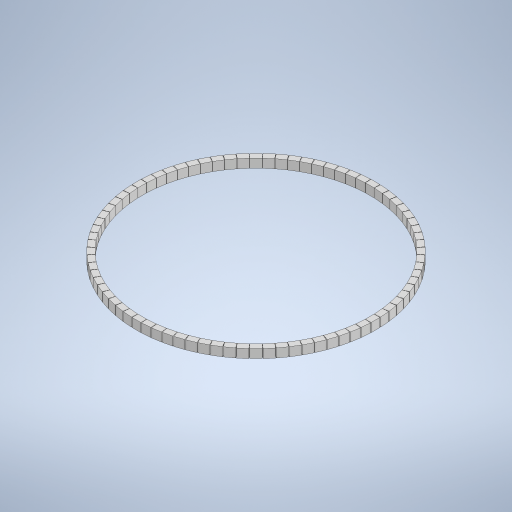
# Autodesk Inventor part: 屋-2 磚-1
Saved by Autodesk Inventor 2024 (Build 280153000, 153)
## iProperties
Created: 2024-05-21
Part Number: 屋-2 磚-1
Material: 一般
Document SubType Name: Modeling
Designer: User
Density: 1 g/cm^3
Appearance: 預設
Author: User
Autodesk Inventor part; units mm, degrees
ref_plane "YZ Plane" through (0, 0, 0) normal (1, 0, 0) x (0, 1, 0)
ref_plane "XZ Plane" through (0, 0, 0) normal (0, 1, 0) x (-1, 0, 0)
ref_plane "XY Plane" through (0, 0, 0) normal (0, 0, 1) x (1, 0, 0)
sketch "草圖1" plane through (0, 0, 0) normal (0, 1, 0) x (-1, 0, 0)
  circle A0 centre (0, 0) radius 20
  line L0 (19.5, 0.75) -> (20.5, 0.75)
  line L1 (20.5, 0.75) -> (20.5, -0.75)
  line L2 (20.5, -0.75) -> (19.5, -0.75)
  line L3 (19.5, -0.75) -> (19.5, 0.75)
  line L4 (19.5, 0.75) -> (20.5, -0.75) construction
  line L5 (20.5, 0.75) -> (19.5, -0.75) construction
  line L6 (20.378, 2.3561) -> (20.4956, 0.8607)
  line L7 (20.4956, 0.8607) -> (19.4987, 0.7823)
  line L8 (19.4987, 0.7823) -> (19.381, 2.2776)
  line L9 (19.381, 2.2776) -> (20.378, 2.3561)
  line L10 (20.1303, 3.9477) -> (20.3649, 2.4661)
  line L11 (20.3649, 2.4661) -> (19.3772, 2.3097)
  line L12 (19.3772, 2.3097) -> (19.1426, 3.7912)
  line L13 (19.1426, 3.7912) -> (20.1303, 3.9477)
  line L14 (19.7585, 5.5149) -> (20.1087, 4.0564)
  line L15 (20.1087, 4.0564) -> (19.1363, 3.8229)
  line L16 (19.1363, 3.8229) -> (18.7861, 5.2815)
  line L17 (18.7861, 5.2815) -> (19.7585, 5.5149)
  line L18 (19.2649, 7.0481) -> (19.7284, 5.6216)
  line L19 (19.7284, 5.6216) -> (18.7774, 5.3125)
  line L20 (18.7774, 5.3125) -> (18.3138, 6.7391)
  line L21 (18.3138, 6.7391) -> (19.2649, 7.0481)
  line L22 (18.6525, 8.5379) -> (19.2265, 7.1521)
  line L23 (19.2265, 7.1521) -> (18.3027, 6.7694)
  line L24 (18.3027, 6.7694) -> (17.7286, 8.1552)
  line L25 (17.7286, 8.1552) -> (18.6525, 8.5379)
  line L26 (17.9251, 9.9751) -> (18.6061, 8.6386)
  line L27 (18.6061, 8.6386) -> (17.7151, 8.1846)
  line L28 (17.7151, 8.1846) -> (17.0341, 9.5211)
  line L29 (17.0341, 9.5211) -> (17.9251, 9.9751)
  line L30 (17.0872, 11.3507) -> (17.871, 10.0717)
  line L31 (17.871, 10.0717) -> (17.0184, 9.5492)
  line L32 (17.0184, 9.5492) -> (16.2346, 10.8282)
  line L33 (16.2346, 10.8282) -> (17.0872, 11.3507)
  line L34 (16.144, 12.6564) -> (17.0257, 11.4428)
  line L35 (17.0257, 11.4428) -> (16.2167, 10.855)
  line L36 (16.2167, 10.855) -> (15.335, 12.0686)
  line L37 (15.335, 12.0686) -> (16.144, 12.6564)
  line L38 (15.1012, 13.884) -> (16.0754, 12.7434)
  line L39 (16.0754, 12.7434) -> (15.315, 12.0939)
  line L40 (15.315, 12.0939) -> (14.3408, 13.2345)
  line L41 (14.3408, 13.2345) -> (15.1012, 13.884)
  line L42 (13.9654, 15.026) -> (15.026, 13.9654)
  line L43 (15.026, 13.9654) -> (14.3189, 13.2583)
  line L44 (14.3189, 13.2583) -> (13.2583, 14.3189)
  line L45 (13.2583, 14.3189) -> (13.9654, 15.026)
  line L46 (12.7434, 16.0754) -> (13.884, 15.1012)
  line L47 (13.884, 15.1012) -> (13.2345, 14.3408)
  line L48 (13.2345, 14.3408) -> (12.0939, 15.315)
  line L49 (12.0939, 15.315) -> (12.7434, 16.0754)
  line L50 (11.4428, 17.0257) -> (12.6564, 16.144)
  line L51 (12.6564, 16.144) -> (12.0686, 15.335)
  line L52 (12.0686, 15.335) -> (10.855, 16.2167)
  line L53 (10.855, 16.2167) -> (11.4428, 17.0257)
  line L54 (10.0717, 17.871) -> (11.3507, 17.0872)
  line L55 (11.3507, 17.0872) -> (10.8282, 16.2346)
  line L56 (10.8282, 16.2346) -> (9.5492, 17.0184)
  line L57 (9.5492, 17.0184) -> (10.0717, 17.871)
  line L58 (8.6386, 18.6061) -> (9.9751, 17.9251)
  line L59 (9.9751, 17.9251) -> (9.5211, 17.0341)
  line L60 (9.5211, 17.0341) -> (8.1846, 17.7151)
  line L61 (8.1846, 17.7151) -> (8.6386, 18.6061)
  line L62 (7.1521, 19.2265) -> (8.5379, 18.6525)
  line L63 (8.5379, 18.6525) -> (8.1552, 17.7286)
  line L64 (8.1552, 17.7286) -> (6.7694, 18.3027)
  line L65 (6.7694, 18.3027) -> (7.1521, 19.2265)
  line L66 (5.6216, 19.7284) -> (7.0481, 19.2649)
  line L67 (7.0481, 19.2649) -> (6.7391, 18.3138)
  line L68 (6.7391, 18.3138) -> (5.3125, 18.7774)
  line L69 (5.3125, 18.7774) -> (5.6216, 19.7284)
  line L70 (4.0564, 20.1087) -> (5.5149, 19.7585)
  line L71 (5.5149, 19.7585) -> (5.2815, 18.7861)
  line L72 (5.2815, 18.7861) -> (3.8229, 19.1363)
  line L73 (3.8229, 19.1363) -> (4.0564, 20.1087)
  line L74 (2.4661, 20.3649) -> (3.9477, 20.1303)
  line L75 (3.9477, 20.1303) -> (3.7912, 19.1426)
  line L76 (3.7912, 19.1426) -> (2.3097, 19.3772)
  line L77 (2.3097, 19.3772) -> (2.4661, 20.3649)
  line L78 (0.8607, 20.4956) -> (2.3561, 20.378)
  line L79 (2.3561, 20.378) -> (2.2776, 19.381)
  line L80 (2.2776, 19.381) -> (0.7823, 19.4987)
  line L81 (0.7823, 19.4987) -> (0.8607, 20.4956)
  line L82 (-0.75, 20.5) -> (0.75, 20.5)
  line L83 (0.75, 20.5) -> (0.75, 19.5)
  line L84 (0.75, 19.5) -> (-0.75, 19.5)
  line L85 (-0.75, 19.5) -> (-0.75, 20.5)
  line L86 (-2.3561, 20.378) -> (-0.8607, 20.4956)
  line L87 (-0.8607, 20.4956) -> (-0.7823, 19.4987)
  line L88 (-0.7823, 19.4987) -> (-2.2776, 19.381)
  line L89 (-2.2776, 19.381) -> (-2.3561, 20.378)
  line L90 (-3.9477, 20.1303) -> (-2.4661, 20.3649)
  line L91 (-2.4661, 20.3649) -> (-2.3097, 19.3772)
  line L92 (-2.3097, 19.3772) -> (-3.7912, 19.1426)
  line L93 (-3.7912, 19.1426) -> (-3.9477, 20.1303)
  line L94 (-5.5149, 19.7585) -> (-4.0564, 20.1087)
  line L95 (-4.0564, 20.1087) -> (-3.8229, 19.1363)
  line L96 (-3.8229, 19.1363) -> (-5.2815, 18.7861)
  line L97 (-5.2815, 18.7861) -> (-5.5149, 19.7585)
  line L98 (-7.0481, 19.2649) -> (-5.6216, 19.7284)
  line L99 (-5.6216, 19.7284) -> (-5.3125, 18.7774)
  line L100 (-5.3125, 18.7774) -> (-6.7391, 18.3138)
  line L101 (-6.7391, 18.3138) -> (-7.0481, 19.2649)
  line L102 (-8.5379, 18.6525) -> (-7.1521, 19.2265)
  line L103 (-7.1521, 19.2265) -> (-6.7694, 18.3027)
  line L104 (-6.7694, 18.3027) -> (-8.1552, 17.7286)
  line L105 (-8.1552, 17.7286) -> (-8.5379, 18.6525)
  line L106 (-9.9751, 17.9251) -> (-8.6386, 18.6061)
  line L107 (-8.6386, 18.6061) -> (-8.1846, 17.7151)
  line L108 (-8.1846, 17.7151) -> (-9.5211, 17.0341)
  line L109 (-9.5211, 17.0341) -> (-9.9751, 17.9251)
  line L110 (-11.3507, 17.0872) -> (-10.0717, 17.871)
  line L111 (-10.0717, 17.871) -> (-9.5492, 17.0184)
  line L112 (-9.5492, 17.0184) -> (-10.8282, 16.2346)
  line L113 (-10.8282, 16.2346) -> (-11.3507, 17.0872)
  line L114 (-12.6564, 16.144) -> (-11.4428, 17.0257)
  line L115 (-11.4428, 17.0257) -> (-10.855, 16.2167)
  line L116 (-10.855, 16.2167) -> (-12.0686, 15.335)
  line L117 (-12.0686, 15.335) -> (-12.6564, 16.144)
  line L118 (-13.884, 15.1012) -> (-12.7434, 16.0754)
  line L119 (-12.7434, 16.0754) -> (-12.0939, 15.315)
  line L120 (-12.0939, 15.315) -> (-13.2345, 14.3408)
  line L121 (-13.2345, 14.3408) -> (-13.884, 15.1012)
  line L122 (-15.026, 13.9654) -> (-13.9654, 15.026)
  line L123 (-13.9654, 15.026) -> (-13.2583, 14.3189)
  line L124 (-13.2583, 14.3189) -> (-14.3189, 13.2583)
  line L125 (-14.3189, 13.2583) -> (-15.026, 13.9654)
  line L126 (-16.0754, 12.7434) -> (-15.1012, 13.884)
  line L127 (-15.1012, 13.884) -> (-14.3408, 13.2345)
  line L128 (-14.3408, 13.2345) -> (-15.315, 12.0939)
  line L129 (-15.315, 12.0939) -> (-16.0754, 12.7434)
  line L130 (-17.0257, 11.4428) -> (-16.144, 12.6564)
  line L131 (-16.144, 12.6564) -> (-15.335, 12.0686)
  line L132 (-15.335, 12.0686) -> (-16.2167, 10.855)
  line L133 (-16.2167, 10.855) -> (-17.0257, 11.4428)
  line L134 (-17.871, 10.0717) -> (-17.0872, 11.3507)
  line L135 (-17.0872, 11.3507) -> (-16.2346, 10.8282)
  line L136 (-16.2346, 10.8282) -> (-17.0184, 9.5492)
  line L137 (-17.0184, 9.5492) -> (-17.871, 10.0717)
  line L138 (-18.6061, 8.6386) -> (-17.9251, 9.9751)
  line L139 (-17.9251, 9.9751) -> (-17.0341, 9.5211)
  line L140 (-17.0341, 9.5211) -> (-17.7151, 8.1846)
  line L141 (-17.7151, 8.1846) -> (-18.6061, 8.6386)
  line L142 (-19.2265, 7.1521) -> (-18.6525, 8.5379)
  line L143 (-18.6525, 8.5379) -> (-17.7286, 8.1552)
  line L144 (-17.7286, 8.1552) -> (-18.3027, 6.7694)
  line L145 (-18.3027, 6.7694) -> (-19.2265, 7.1521)
  line L146 (-19.7284, 5.6216) -> (-19.2649, 7.0481)
  line L147 (-19.2649, 7.0481) -> (-18.3138, 6.7391)
  line L148 (-18.3138, 6.7391) -> (-18.7774, 5.3125)
  line L149 (-18.7774, 5.3125) -> (-19.7284, 5.6216)
  line L150 (-20.1087, 4.0564) -> (-19.7585, 5.5149)
  line L151 (-19.7585, 5.5149) -> (-18.7861, 5.2815)
  line L152 (-18.7861, 5.2815) -> (-19.1363, 3.8229)
  line L153 (-19.1363, 3.8229) -> (-20.1087, 4.0564)
  line L154 (-20.3649, 2.4661) -> (-20.1303, 3.9477)
  line L155 (-20.1303, 3.9477) -> (-19.1426, 3.7912)
  line L156 (-19.1426, 3.7912) -> (-19.3772, 2.3097)
  line L157 (-19.3772, 2.3097) -> (-20.3649, 2.4661)
  line L158 (-20.4956, 0.8607) -> (-20.378, 2.3561)
  line L159 (-20.378, 2.3561) -> (-19.381, 2.2776)
  line L160 (-19.381, 2.2776) -> (-19.4987, 0.7823)
  line L161 (-19.4987, 0.7823) -> (-20.4956, 0.8607)
  line L162 (-20.5, -0.75) -> (-20.5, 0.75)
  line L163 (-20.5, 0.75) -> (-19.5, 0.75)
  line L164 (-19.5, 0.75) -> (-19.5, -0.75)
  line L165 (-19.5, -0.75) -> (-20.5, -0.75)
  line L166 (-20.378, -2.3561) -> (-20.4956, -0.8607)
  line L167 (-20.4956, -0.8607) -> (-19.4987, -0.7823)
  line L168 (-19.4987, -0.7823) -> (-19.381, -2.2776)
  line L169 (-19.381, -2.2776) -> (-20.378, -2.3561)
  line L170 (-20.1303, -3.9477) -> (-20.3649, -2.4661)
  line L171 (-20.3649, -2.4661) -> (-19.3772, -2.3097)
  line L172 (-19.3772, -2.3097) -> (-19.1426, -3.7912)
  line L173 (-19.1426, -3.7912) -> (-20.1303, -3.9477)
  line L174 (-19.7585, -5.5149) -> (-20.1087, -4.0564)
  line L175 (-20.1087, -4.0564) -> (-19.1363, -3.8229)
  line L176 (-19.1363, -3.8229) -> (-18.7861, -5.2815)
  line L177 (-18.7861, -5.2815) -> (-19.7585, -5.5149)
  line L178 (-19.2649, -7.0481) -> (-19.7284, -5.6216)
  line L179 (-19.7284, -5.6216) -> (-18.7774, -5.3125)
  line L180 (-18.7774, -5.3125) -> (-18.3138, -6.7391)
  line L181 (-18.3138, -6.7391) -> (-19.2649, -7.0481)
  line L182 (-18.6525, -8.5379) -> (-19.2265, -7.1521)
  line L183 (-19.2265, -7.1521) -> (-18.3027, -6.7694)
  line L184 (-18.3027, -6.7694) -> (-17.7286, -8.1552)
  line L185 (-17.7286, -8.1552) -> (-18.6525, -8.5379)
  line L186 (-17.9251, -9.9751) -> (-18.6061, -8.6386)
  line L187 (-18.6061, -8.6386) -> (-17.7151, -8.1846)
  line L188 (-17.7151, -8.1846) -> (-17.0341, -9.5211)
  line L189 (-17.0341, -9.5211) -> (-17.9251, -9.9751)
  line L190 (-17.0872, -11.3507) -> (-17.871, -10.0717)
  line L191 (-17.871, -10.0717) -> (-17.0184, -9.5492)
  line L192 (-17.0184, -9.5492) -> (-16.2346, -10.8282)
  line L193 (-16.2346, -10.8282) -> (-17.0872, -11.3507)
  line L194 (-16.144, -12.6564) -> (-17.0257, -11.4428)
  line L195 (-17.0257, -11.4428) -> (-16.2167, -10.855)
  line L196 (-16.2167, -10.855) -> (-15.335, -12.0686)
  line L197 (-15.335, -12.0686) -> (-16.144, -12.6564)
  line L198 (-15.1012, -13.884) -> (-16.0754, -12.7434)
  line L199 (-16.0754, -12.7434) -> (-15.315, -12.0939)
  line L200 (-15.315, -12.0939) -> (-14.3408, -13.2345)
  line L201 (-14.3408, -13.2345) -> (-15.1012, -13.884)
  line L202 (-13.9654, -15.026) -> (-15.026, -13.9654)
  line L203 (-15.026, -13.9654) -> (-14.3189, -13.2583)
  line L204 (-14.3189, -13.2583) -> (-13.2583, -14.3189)
  line L205 (-13.2583, -14.3189) -> (-13.9654, -15.026)
  line L206 (-12.7434, -16.0754) -> (-13.884, -15.1012)
  line L207 (-13.884, -15.1012) -> (-13.2345, -14.3408)
  line L208 (-13.2345, -14.3408) -> (-12.0939, -15.315)
  line L209 (-12.0939, -15.315) -> (-12.7434, -16.0754)
  line L210 (-11.4428, -17.0257) -> (-12.6564, -16.144)
  line L211 (-12.6564, -16.144) -> (-12.0686, -15.335)
  line L212 (-12.0686, -15.335) -> (-10.855, -16.2167)
  line L213 (-10.855, -16.2167) -> (-11.4428, -17.0257)
  line L214 (-10.0717, -17.871) -> (-11.3507, -17.0872)
  line L215 (-11.3507, -17.0872) -> (-10.8282, -16.2346)
  line L216 (-10.8282, -16.2346) -> (-9.5492, -17.0184)
  line L217 (-9.5492, -17.0184) -> (-10.0717, -17.871)
  line L218 (-8.6386, -18.6061) -> (-9.9751, -17.9251)
  line L219 (-9.9751, -17.9251) -> (-9.5211, -17.0341)
  line L220 (-9.5211, -17.0341) -> (-8.1846, -17.7151)
  line L221 (-8.1846, -17.7151) -> (-8.6386, -18.6061)
  line L222 (-7.1521, -19.2265) -> (-8.5379, -18.6525)
  line L223 (-8.5379, -18.6525) -> (-8.1552, -17.7286)
  line L224 (-8.1552, -17.7286) -> (-6.7694, -18.3027)
  line L225 (-6.7694, -18.3027) -> (-7.1521, -19.2265)
  line L226 (-5.6216, -19.7284) -> (-7.0481, -19.2649)
  line L227 (-7.0481, -19.2649) -> (-6.7391, -18.3138)
  line L228 (-6.7391, -18.3138) -> (-5.3125, -18.7774)
  line L229 (-5.3125, -18.7774) -> (-5.6216, -19.7284)
  line L230 (-4.0564, -20.1087) -> (-5.5149, -19.7585)
  line L231 (-5.5149, -19.7585) -> (-5.2815, -18.7861)
  line L232 (-5.2815, -18.7861) -> (-3.8229, -19.1363)
  line L233 (-3.8229, -19.1363) -> (-4.0564, -20.1087)
  line L234 (-2.4661, -20.3649) -> (-3.9477, -20.1303)
  line L235 (-3.9477, -20.1303) -> (-3.7912, -19.1426)
  line L236 (-3.7912, -19.1426) -> (-2.3097, -19.3772)
  line L237 (-2.3097, -19.3772) -> (-2.4661, -20.3649)
  line L238 (-0.8607, -20.4956) -> (-2.3561, -20.378)
  line L239 (-2.3561, -20.378) -> (-2.2776, -19.381)
  line L240 (-2.2776, -19.381) -> (-0.7823, -19.4987)
  line L241 (-0.7823, -19.4987) -> (-0.8607, -20.4956)
  line L242 (0.75, -20.5) -> (-0.75, -20.5)
  line L243 (-0.75, -20.5) -> (-0.75, -19.5)
  line L244 (-0.75, -19.5) -> (0.75, -19.5)
  line L245 (0.75, -19.5) -> (0.75, -20.5)
  line L246 (2.3561, -20.378) -> (0.8607, -20.4956)
  line L247 (0.8607, -20.4956) -> (0.7823, -19.4987)
  line L248 (0.7823, -19.4987) -> (2.2776, -19.381)
  line L249 (2.2776, -19.381) -> (2.3561, -20.378)
  line L250 (3.9477, -20.1303) -> (2.4661, -20.3649)
  line L251 (2.4661, -20.3649) -> (2.3097, -19.3772)
  line L252 (2.3097, -19.3772) -> (3.7912, -19.1426)
  line L253 (3.7912, -19.1426) -> (3.9477, -20.1303)
  line L254 (5.5149, -19.7585) -> (4.0564, -20.1087)
  line L255 (4.0564, -20.1087) -> (3.8229, -19.1363)
  line L256 (3.8229, -19.1363) -> (5.2815, -18.7861)
  line L257 (5.2815, -18.7861) -> (5.5149, -19.7585)
  line L258 (7.0481, -19.2649) -> (5.6216, -19.7284)
  line L259 (5.6216, -19.7284) -> (5.3125, -18.7774)
  line L260 (5.3125, -18.7774) -> (6.7391, -18.3138)
  line L261 (6.7391, -18.3138) -> (7.0481, -19.2649)
  line L262 (8.5379, -18.6525) -> (7.1521, -19.2265)
  line L263 (7.1521, -19.2265) -> (6.7694, -18.3027)
  line L264 (6.7694, -18.3027) -> (8.1552, -17.7286)
  line L265 (8.1552, -17.7286) -> (8.5379, -18.6525)
  line L266 (9.9751, -17.9251) -> (8.6386, -18.6061)
  line L267 (8.6386, -18.6061) -> (8.1846, -17.7151)
  line L268 (8.1846, -17.7151) -> (9.5211, -17.0341)
  line L269 (9.5211, -17.0341) -> (9.9751, -17.9251)
  line L270 (11.3507, -17.0872) -> (10.0717, -17.871)
  line L271 (10.0717, -17.871) -> (9.5492, -17.0184)
  line L272 (9.5492, -17.0184) -> (10.8282, -16.2346)
  line L273 (10.8282, -16.2346) -> (11.3507, -17.0872)
  line L274 (12.6564, -16.144) -> (11.4428, -17.0257)
  line L275 (11.4428, -17.0257) -> (10.855, -16.2167)
  line L276 (10.855, -16.2167) -> (12.0686, -15.335)
  line L277 (12.0686, -15.335) -> (12.6564, -16.144)
  line L278 (13.884, -15.1012) -> (12.7434, -16.0754)
  line L279 (12.7434, -16.0754) -> (12.0939, -15.315)
  line L280 (12.0939, -15.315) -> (13.2345, -14.3408)
  line L281 (13.2345, -14.3408) -> (13.884, -15.1012)
  line L282 (15.026, -13.9654) -> (13.9654, -15.026)
  line L283 (13.9654, -15.026) -> (13.2583, -14.3189)
  line L284 (13.2583, -14.3189) -> (14.3189, -13.2583)
  line L285 (14.3189, -13.2583) -> (15.026, -13.9654)
  line L286 (16.0754, -12.7434) -> (15.1012, -13.884)
  line L287 (15.1012, -13.884) -> (14.3408, -13.2345)
  line L288 (14.3408, -13.2345) -> (15.315, -12.0939)
  line L289 (15.315, -12.0939) -> (16.0754, -12.7434)
  line L290 (17.0257, -11.4428) -> (16.144, -12.6564)
  line L291 (16.144, -12.6564) -> (15.335, -12.0686)
  line L292 (15.335, -12.0686) -> (16.2167, -10.855)
  line L293 (16.2167, -10.855) -> (17.0257, -11.4428)
  line L294 (17.871, -10.0717) -> (17.0872, -11.3507)
  line L295 (17.0872, -11.3507) -> (16.2346, -10.8282)
  line L296 (16.2346, -10.8282) -> (17.0184, -9.5492)
  line L297 (17.0184, -9.5492) -> (17.871, -10.0717)
  line L298 (18.6061, -8.6386) -> (17.9251, -9.9751)
  line L299 (17.9251, -9.9751) -> (17.0341, -9.5211)
  line L300 (17.0341, -9.5211) -> (17.7151, -8.1846)
  line L301 (17.7151, -8.1846) -> (18.6061, -8.6386)
  line L302 (19.2265, -7.1521) -> (18.6525, -8.5379)
  line L303 (18.6525, -8.5379) -> (17.7286, -8.1552)
  line L304 (17.7286, -8.1552) -> (18.3027, -6.7694)
  line L305 (18.3027, -6.7694) -> (19.2265, -7.1521)
  line L306 (19.7284, -5.6216) -> (19.2649, -7.0481)
  line L307 (19.2649, -7.0481) -> (18.3138, -6.7391)
  line L308 (18.3138, -6.7391) -> (18.7774, -5.3125)
  line L309 (18.7774, -5.3125) -> (19.7284, -5.6216)
  line L310 (20.1087, -4.0564) -> (19.7585, -5.5149)
  line L311 (19.7585, -5.5149) -> (18.7861, -5.2815)
  line L312 (18.7861, -5.2815) -> (19.1363, -3.8229)
  line L313 (19.1363, -3.8229) -> (20.1087, -4.0564)
  line L314 (20.3649, -2.4661) -> (20.1303, -3.9477)
  line L315 (20.1303, -3.9477) -> (19.1426, -3.7912)
  line L316 (19.1426, -3.7912) -> (19.3772, -2.3097)
  line L317 (19.3772, -2.3097) -> (20.3649, -2.4661)
  line L318 (20.4956, -0.8607) -> (20.378, -2.3561)
  line L319 (20.378, -2.3561) -> (19.381, -2.2776)
  line L320 (19.381, -2.2776) -> (19.4987, -0.7823)
  line L321 (19.4987, -0.7823) -> (20.4956, -0.8607)
  point P0 (20, 0)
  dimension "d0" = 40
  dimension "d1" = 1
  dimension "d2" = 1.5
  dimension "d5" = 360
  constraints: 644 end point, 2 midpoint, 2 parallel, 1 coincident, 1 horizontal, 1 horizontal alignment, 1 perpendicular, 643 other
  measures "d1" distance of L1.end L2.end
  measures "d2" distance of L0.end L1.end
extrude "擠出1" add sketch "草圖1" along normal blind 1.5 contours A0 L2 L3 L0 | A0 L0 L1 L2 | L7 L8 L9 A0 | A0 L9 L6 L7 | L321 L318 L319 A0 | A0 L319 L320 L321 | L11 L12 L13 A0 | A0 L13 L10 L11 | L317 L314 L315 A0 | A0 L315 L316 L317 | L15 L16 L17 A0 | A0 L17 L14 L15 | L313 L310 L311 A0 | A0 L311 L312 L313 | L19 L20 L21 A0 | A0 L21 L18 L19 | L309 L306 L307 A0 | A0 L307 L308 L309 | L23 L24 L25 A0 | A0 L25 L22 L23 | L305 L302 L303 A0 | A0 L303 L304 L305 | L27 L28 L29 A0 | A0 L29 L26 L27 | L301 L298 L299 A0 | A0 L299 L300 L301 | L31 L32 L33 A0 | A0 L33 L30 L31 | L297 L294 L295 A0 | A0 L295 L296 L297 | L35 L36 L37 A0 | A0 L37 L34 L35 | L293 L290 L291 A0 | A0 L291 L292 L293 | L39 L40 L41 A0 | A0 L41 L38 L39 | L289 L286 L287 A0 | A0 L287 L288 L289 | L43 L44 L45 A0 | A0 L45 L42 L43 | L285 L282 L283 A0 | A0 L283 L284 L285 | L47 L48 L49 A0 | A0 L49 L46 L47 | L281 L278 L279 A0 | A0 L279 L280 L281 | L51 L52 L53 A0 | A0 L53 L50 L51 | L277 L274 L275 A0 | A0 L275 L276 L277 | L55 L56 L57 A0 | A0 L57 L54 L55 | L273 L270 L271 A0 | A0 L271 L272 L273 | L59 L60 L61 A0 | A0 L61 L58 L59 | L269 L266 L267 A0 | A0 L267 L268 L269 | L63 L64 L65 A0 | A0 L65 L62 L63 | L265 L262 L263 A0 | A0 L263 L264 L265 | L67 L68 L69 A0 | A0 L69 L66 L67 | L261 L258 L259 A0 | A0 L259 L260 L261 | L71 L72 L73 A0 | A0 L73 L70 L71 | L257 L254 L255 A0 | A0 L255 L256 L257 | L75 L76 L77 A0 | A0 L77 L74 L75 | L253 L250 L251 A0 | A0 L251 L252 L253 | L79 L80 L81 A0 | A0 L81 L78 L79 | L249 L246 L247 A0 | A0 L247 L248 L249 | L83 L84 L85 A0 | A0 L85 L82 L83 | L245 L242 L243 A0 | A0 L243 L244 L245 | L87 L88 L89 A0 | A0 L89 L86 L87 | L241 L238 L239 A0 | A0 L239 L240 L241 | L91 L92 L93 A0 | A0 L93 L90 L91 | L237 L234 L235 A0 | A0 L235 L236 L237 | L95 L96 L97 A0 | A0 L97 L94 L95 | L233 L230 L231 A0 | A0 L231 L232 L233 | L99 L100 L101 A0 | A0 L101 L98 L99 | L229 L226 L227 A0 | A0 L227 L228 L229 | L103 L104 L105 A0 | A0 L105 L102 L103 | L225 L222 L223 A0 | A0 L223 L224 L225 | L107 L108 L109 A0 | A0 L109 L106 L107 | L221 L218 L219 A0 | A0 L219 L220 L221 | L111 L112 L113 A0 | A0 L113 L110 L111 | L217 L214 L215 A0 | A0 L215 L216 L217 | L115 L116 L117 A0 | A0 L117 L114 L115 | L213 L210 L211 A0 | A0 L211 L212 L213 | L119 L120 L121 A0 | A0 L121 L118 L119 | L209 L206 L207 A0 | A0 L207 L208 L209 | L123 L124 L125 A0 | A0 L125 L122 L123 | L205 L202 L203 A0 | A0 L203 L204 L205 | L127 L128 L129 A0 | A0 L129 L126 L127 | L201 L198 L199 A0 | A0 L199 L200 L201 | L131 L132 L133 A0 | A0 L133 L130 L131 | L197 L194 L195 A0 | A0 L195 L196 L197 | L135 L136 L137 A0 | A0 L137 L134 L135 | L193 L190 L191 A0 | A0 L191 L192 L193 | L139 L140 L141 A0 | A0 L141 L138 L139 | L189 L186 L187 A0 | A0 L187 L188 L189 | L143 L144 L145 A0 | A0 L145 L142 L143 | L185 L182 L183 A0 | A0 L183 L184 L185 | L147 L148 L149 A0 | A0 L149 L146 L147 | L181 L178 L179 A0 | A0 L179 L180 L181 | L151 L152 L153 A0 | A0 L153 L150 L151 | L177 L174 L175 A0 | A0 L175 L176 L177 | L155 L156 L157 A0 | A0 L157 L154 L155 | L173 L170 L171 A0 | A0 L171 L172 L173 | L159 L160 L161 A0 | A0 L161 L158 L159 | L169 L166 L167 A0 | A0 L167 L168 L169 | L163 L164 L165 A0 | A0 L165 L162 L163
sketch "草圖2" plane through (0, 1.5, 0) normal (0, 1, 0) x (1, 0, 0)
  circle A0 centre (0, 0) radius 20.05
  circle A1 centre (0, 0) radius 19.95
  dimension "d9" = 40.1
  dimension "d10" = 39.9
  constraints: 2 centre point, 2 coincident
  measures "d9" diameter of A0
  measures "d10" diameter of A1
extrude "擠出2" add sketch "草圖2" against normal blind 1.5
